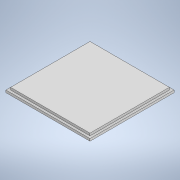
# Autodesk Inventor part: lid
Saved by Autodesk Inventor 2020 (Build 240168000, 168)
## iProperties
Created: 2020-01-15
Part Number: lid
Material: Generic
Document SubType Name: Modeling
Designer: ColinP
Density: 1 g/cm^3
Appearance: Default
Author: ColinP
Autodesk Inventor part; units mm, degrees
ref_plane "YZ Plane" through (0, 0, 0) normal (1, 0, 0) x (0, 1, 0)
ref_plane "XZ Plane" through (0, 0, 0) normal (0, 1, 0) x (-1, 0, 0)
ref_plane "XY Plane" through (0, 0, 0) normal (0, 0, 1) x (1, 0, 0)
sketch "Sketch1" plane through (0, 0, 0) normal (0, 1, 0) x (-1, 0, 0)
  line L0 (0, 0) -> (-114.3, 0)
  line L1 (0, 0) -> (114.3, 0) construction
  line L2 (-114.3, 0) -> (-114.3, -114.3)
  line L3 (-114.3, -114.3) -> (114.3, -114.3)
  line L4 (114.3, -114.3) -> (114.3, 114.3)
  line L5 (114.3, 114.3) -> (-114.3, 114.3)
  line L6 (-114.3, 114.3) -> (-114.3, 0)
  line L7 (114.3, 114.3) -> (114.3, 107.95)
  line L8 (114.3, 107.95) -> (107.95, 107.95)
  line L9 (107.95, 107.95) -> (107.95, -107.95)
  line L10 (107.95, -107.95) -> (-107.95, -107.95)
  line L11 (-107.95, -107.95) -> (-107.95, 107.95)
  line L12 (-107.95, 107.95) -> (107.95, 107.95)
  dimension "d0" = 114.3
  dimension "d1" = 180
  dimension "d2" = 114.3
  dimension "d3" = 228.6
  dimension "d4" = 228.6
  dimension "d5" = 6.35
  dimension "d6" = 6.35
  dimension "d7" = 215.9
  dimension "d8" = 215.9
  dimension "d9" = 215.9
  constraints: 26 end point, 7 perpendicular, 3 point on line, 2 collinear, 2 horizontal
  measures "d0" distance of L0.start L0.end
  measures "d1" angle of L0 L1
  measures "d2" distance of L0.end L2.end
  measures "d3" distance of L2.end L3.end
  measures "d4" distance of L3.end L4.end
  measures "d5" distance of L4.end L7.end
  measures "d6" distance of L7.end L8.end
  measures "d7" distance of L8.end L9.end
  measures "d8" distance of L9.end L10.end
  measures "d9" distance of L10.end L11.end
extrude "Extrusion1" add sketch "Sketch1" along normal blind 6.35
extrude "Extrusion2" add sketch "Sketch1" along normal blind 12.7 contours L11 L12 L9 L10
body "Solid1"
